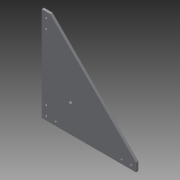
# Autodesk Inventor part: GUSSET_200MM
Saved by Autodesk Inventor 2013 (Build 170138000, 138)
## iProperties
Created: 2013-06-20
Part Number: GUSSET_200MM
Material: Generic
Document SubType Name: Modeling
Designer: Brett
Density: 1 g/cm^3
Author: Brett
Autodesk Inventor part; units mm, degrees
ref_plane "YZ Plane" through (0, 0, 0) normal (1, 0, 0) x (0, 1, 0)
ref_plane "XZ Plane" through (0, 0, 0) normal (0, 1, 0) x (-1, 0, 0)
ref_plane "XY Plane" through (0, 0, 0) normal (0, 0, 1) x (1, 0, 0)
sketch "Sketch1" plane through (0, 0, 0) normal (0, 0, 1) x (1, 0, 0)
  circle A0 centre (9, 9) radius 2.5
  line L0 (200, 18) -> (200, 0)
  line L1 (200, 0) -> (0, 0)
  line L2 (0, 0) -> (0, 200)
  line L3 (0, 200) -> (18, 200)
  line L4 (18, 200) -> (200, 18)
  circle A1 centre (29, 9) radius 2.5
  circle A2 centre (169, 9) radius 2.5
  circle A3 centre (189, 9) radius 2.5
  circle A4 centre (9, 29) radius 2.5
  circle A5 centre (9, 169) radius 2.5
  circle A6 centre (9, 189) radius 2.5
  constraints: 10 end point, 7 centre point, 6 equal radius, 2 perpendicular, 1 parallel
extrude "Extrusion1" add sketch "Sketch1" along normal blind 5
hole "Hole1" at (60, 60, 5) direction (0, 0, -1) diameter 7.75 end through all
body "Solid1"
